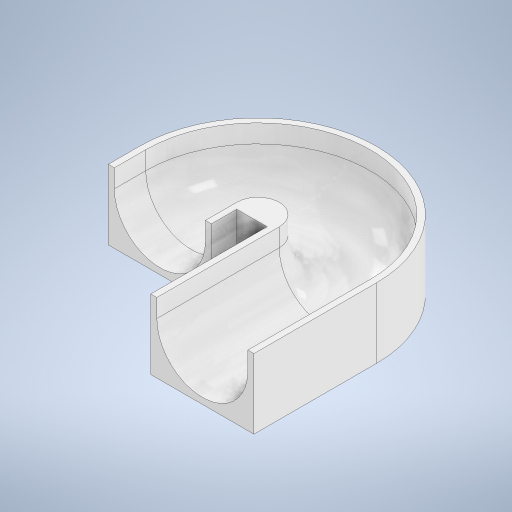
# Autodesk Inventor part: Troca de sentido
Saved by Autodesk Inventor 2024 (Build 280153000, 153)
## iProperties
Created: 2023-05-09
Part Number: Troca de sentido
Material: Plástico PET
Document SubType Name: Modeling
Designer: jpjoa
Density: 1.541 g/cm^3
Appearance: Branco
Author: jpjoa
Autodesk Inventor part; units mm, degrees
ref_plane "YZ Plane" through (0, 0, 0) normal (1, 0, 0) x (0, 1, 0)
ref_plane "XZ Plane" through (0, 0, 0) normal (0, 1, 0) x (-1, 0, 0)
ref_plane "XY Plane" through (0, 0, 0) normal (0, 0, 1) x (1, 0, 0)
sketch "Esboço1" plane through (0, 0, 0) normal (0, 1, 0) x (-1, 0, 0)
  line L0 (-1.2, -1.2) -> (-19.2, -1.2)
  line L1 (-19.2, -1.2) -> (-19.2, -6.2)
  line L2 (-19.2, -6.2) -> (-27.6, -6.2)
  line L3 (-27.6, -6.2) -> (-27.6, -1.2)
  line L4 (-27.6, -1.2) -> (-45.6, -1.2)
  line L5 (-45.6, -1.2) -> (-45.6, -6.2)
  arc A0 (-45.6, -6.2) -> (-1.2, -6.2) centre (-23.4, -6.2) ccw
  line L6 (-23.4, -6.2) -> (-45.6, -6.2) construction
  line L7 (-23.4, -6.2) -> (-1.2, -6.2) construction
  line L8 (-1.2, -6.2) -> (-1.2, -1.2)
  arc A1 (-46.8, -6.2) -> (0, -6.2) centre (-23.4, -6.2) ccw
  line L9 (0, -6.2) -> (0, 0)
  line L10 (0, 0) -> (-20.4, 0)
  line L11 (-20.4, 0) -> (-20.4, -5)
  line L12 (-20.4, -5) -> (-26.4, -5)
  line L13 (-46.8, 18) -> (-46.8, -6.2)
  line L14 (-27.6, -1.2) -> (-27.6, 18)
  line L15 (-19.2, -1.2) -> (-19.2, 0)
  line L16 (-1.2, -1.2) -> (-1.2, 0)
  arc A2 (-27.6, -6.2) -> (-19.2, -6.2) centre (-23.4, -6.2) ccw
  line L17 (-26.4, 18) -> (-46.8, 18)
  line L18 (-45.6, -1.2) -> (-45.6, 18)
  line L19 (-26.4, 18) -> (-26.4, -5)
  point P0 (-23.4, -6.2)
  point P1 (-46.8, -6.2)
  point P2 (-19.2, -6.2)
  point P3 (-27.6, -6.2)
  point P4 (-45.6, -6.2)
  point P5 (-36.6, 18)
  point P6 (-36.6, -1.2)
  point P7 (-45.6, -3.7)
  point P8 (-45.6, 8.4)
  point P9 (-23.4, -5)
  point P10 (-26.4, 6.5)
  dimension "d0" = 18
  dimension "d1" = 180
  dimension "d3" = 1.2
  dimension "d7" = 18
  dimension "d15" = 1.2
  dimension "d16" = 6
  dimension "d18" = 19.2
  dimension "d19" = 5
  constraints: 40 end point, 12 coincident, 10 perpendicular, 8 horizontal alignment, 7 midpoint, 6 point on circle, 4 point on line, 3 centre point, 3 vertical alignment, 2 horizontal, 2 vertical, 1 collinear, 4 other
  measures "d0" distance of L0.start L0.end
  measures "d1" angle of L7 L6
  measures "d3" radial gap between concentric circles of A0 A1
  measures "d7" radial gap between concentric circles of A0 A2
  measures "d15" distance between parallel lines of L3 L19
  measures "d16" distance between parallel lines of L11 L19
  measures "d18" distance of L18.start L18.end
  measures "d19" distance between parallel lines of L10 L12
extrude "Extrusão1" add sketch "Esboço1" against normal blind 1.2
extrude "Extrusão3" add sketch "Esboço1" along normal blind 12.6 contours L16 L10 L9 A1 L13 L17 L18 L5 A0 L8 | L1 L2 L3 L14 L17 L19 L12 L11 L10 L15 | A2 L2
fillet "Arredondamento1" radius 9 6 edges at (1.2, 0, -3.1) (45.6, 0, 5.9) (23.4, 0, -28.4) (27.6, 0, 5.9) (19.2, 0, -3.1) (23.4, 0, -10.4)
equation "\"d0\" = Diâmetro_esfera"
equation "\"d3\" = Margem"
equation "\"d15\" = Margem"
equation "\"d16\" = Espessura_torre_base"
equation "\"d8\" = Margem"
equation "\"d12\" = 0.7 * Diâmetro_esfera"
equation "\"d14\" = 0.5 * Diâmetro_esfera"
equation "\"Diâmetro_esfera\" = 18"
equation "\"Filamento\" = 0.4"
equation "\"Margem\" = 3 * Filamento"
equation "\"Espessura_torre_base\" = 15 * Filamento"
